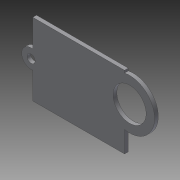
# Autodesk Inventor part: Controller_faceplate_v0.1
Saved by Autodesk Inventor 2015 (Build 190159000, 159)
## iProperties
Created: 2016-02-03
Part Number: Controller_faceplate_v0.1
Material: Generic
Document SubType Name: Modeling
Designer: wcluser
Density: 1 g/cm^3
Appearance: Default
Author: wcluser
Autodesk Inventor part; units mm, degrees
ref_plane "YZ Plane" through (0, 0, 0) normal (1, 0, 0) x (0, 1, 0)
ref_plane "XZ Plane" through (0, 0, 0) normal (0, 1, 0) x (-1, 0, 0)
ref_plane "XY Plane" through (0, 0, 0) normal (0, 0, 1) x (1, 0, 0)
sketch "Sketch1" plane through (0, 0, 0) normal (0, 1, 0) x (-1, 0, 0)
  line L0 (36.75, 29) -> (36.75, 7.0445)
  line L1 (36.75, -29) -> (-36.75, -29)
  line L2 (-36.75, -29) -> (-36.75, -12.0866)
  line L3 (-36.75, 29) -> (36.75, 29)
  line L4 (36.75, 29) -> (-36.75, -29) construction
  line L5 (36.75, -29) -> (-36.75, 29) construction
  line L6 (-36.75, 27.0891) -> (-36.75, 29)
  arc A0 (36.75, -7.6968) -> (36.75, 7.0445) centre (38.1371, -0.3261) ccw
  circle A1 centre (38.1371, -0.3261) radius 3.25
  line L7 (36.75, -7.6968) -> (36.75, -29)
  arc A2 (-36.75, 27.0891) -> (-36.75, -12.0866) centre (-40.7891, 7.5013) ccw
  circle A3 centre (-40.7891, 7.5013) radius 13.25
  point P0 (0, 0)
  dimension "d0" = 58
  dimension "d1" = 73.5
  dimension "d7" = 6.5
  dimension "d8" = 40
  dimension "d9" = 26.5
  constraints: 16 end point, 5 parallel, 4 centre point, 4 point on circle, 2 coincident, 2 midpoint, 2 perpendicular
  measures "d0" distance of L1.end L3.start
  measures "d1" distance of L1.start L1.end
  measures "d7" diameter of A1
  measures "d8" diameter of A2
  measures "d9" diameter of A3
extrude "Extrusion1" add sketch "Sketch1" along normal blind 3
body "Solid2"
